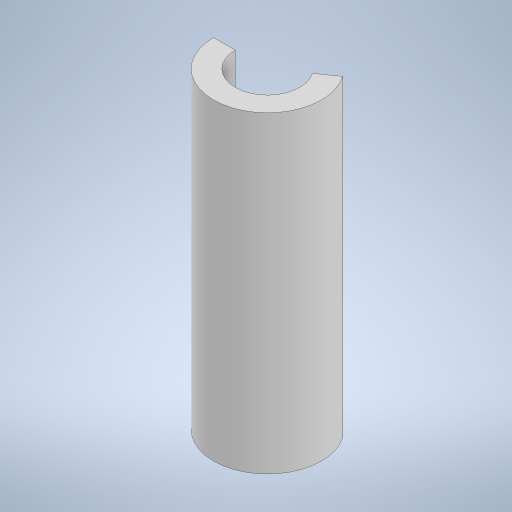
# Autodesk Inventor part: Fuehrung_Taster
Saved by Autodesk Inventor 2023.1 (Build 271208000, 208)
## iProperties
Created: 2023-12-16
Part Number: Fuehrung_Taster
Material: Generisch
Document SubType Name: Modeling
Designer: JansenL
Density: 1 g/cm^3
Appearance: Default
Author: JansenL
Autodesk Inventor part; units mm, degrees
ref_plane "YZ Plane" through (0, 0, 0) normal (1, 0, 0) x (0, 1, 0)
ref_plane "XZ Plane" through (0, 0, 0) normal (0, 1, 0) x (-1, 0, 0)
ref_plane "XY Plane" through (0, 0, 0) normal (0, 0, 1) x (1, 0, 0)
sketch "Sketch2" plane through (0, 0, 0) normal (0, 0, 1) x (1, 0, 0)
  line L0 (-1.85, 0) -> (-1.85, 5)
  line L1 (-1.85, 5) -> (-1.6, 5)
  line L2 (-1.6, 5) -> (-1.6, 13.9)
  line L3 (-1.6, 13.9) -> (-2.675, 13.9)
  line L4 (-2.675, 13.9) -> (-2.675, 0)
  line L5 (-2.675, 0) -> (-1.85, 0)
  line L6 (0, 0) -> (0, 15.301) construction
  line L7 (0, 0) -> (-6.0008, 0) construction
  line L8 (-2.675, 0) -> (-2.675, -1.6)
  line L9 (-2.675, -1.6) -> (-1.85, -1.6)
  line L10 (-1.85, -1.6) -> (-1.85, 0)
  point P0 (-2.2625, -1.6)
  point P1 (-1.85, 0)
  point P2 (-2.675, -0.8)
  dimension "d0" = 1.85
  dimension "d1" = 1.6
  dimension "d2" = 5
  dimension "d3" = 1.6
  dimension "d7" = 13.9
  dimension "d9" = 2.675
  constraints: 22 end point, 6 perpendicular, 3 vertical, 2 collinear, 2 horizontal, 2 midpoint, 1 point on line
  measures "d0" distance between parallel lines of L6 L0
  measures "d1" distance between parallel lines of L6 L2
  measures "d2" distance from line of L6.start L1
  measures "d3" distance from line of L5 point (-2.262, -1.6)
  measures "d7" distance between parallel lines of L5 L3
  measures "d9" distance between parallel lines of L6 L4
revolve "Revolution1" add sketch "Sketch2" angle 215 about axis through (0, 0, 0) along (0, 1, 0)
body "Solid1"
